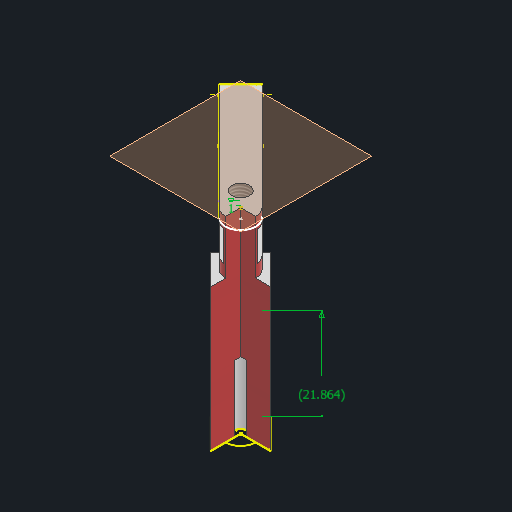
# Autodesk Inventor part: Redesign_Gripper_Finger
Saved by Autodesk Inventor 2025.1 (Build 291241000, 241)
## iProperties
Created: 2024-12-20
Part Number: Redesign_Gripper_Finger
Material: Generic
Document SubType Name: Modeling
Designer: m_kni
Density: 1 g/cm^3
Appearance: Default
Finish1_Area: 560.021 mm^2
Finish1_Appearance: Red
Finish1_Process: Prime/Paint RAL 3018
Finish1_Description: Prime/Paint RAL 3018
Finish1_ShortDescription: RAL 3018
Finish1_Thickness: 0.050 mm
Author: m_kni
## iProperties of the stored document Redesign_Gripper_Finger_3DPrint.ipt
Created: 2025-01-24
Part Number: Redesign_Gripper_Finger_3DPrint
Material: Generic
Document SubType Name: Modeling
Designer: m_kni
Density: 1 g/cm^3
Appearance: Default
Author: m_kni
Autodesk Inventor part; units mm, degrees
ref_plane "YZ Plane" through (0, 0, 0) normal (1, 0, 0) x (0, 1, 0)
ref_plane "XZ Plane" through (0, 0, 0) normal (0, 1, 0) x (-1, 0, 0)
ref_plane "XY Plane" through (0, 0, 0) normal (0, 0, 1) x (1, 0, 0)
sketch "Sketch1" plane through (0, 0, 0) normal (0, 1, 0) x (-1, 0, 0)
  arc A0 (-2.54, 0) -> (0, 2.54) centre (0, 0) ccw
  line L0 (0, 2.54) -> (0, 0)
  line L1 (0, 0) -> (-2.54, 0)
  dimension "d0" = 5.08
  constraints: 4 end point, 2 point on circle, 1 centre point, 1 coincident, 1 perpendicular, 1 vertical
  measures "d0" diameter of A0
extrude "Extrusion1" add sketch "Sketch1" along normal blind 25.4
sketch "Sketch2" plane through (0, 25.4, 0) normal (0, 1, 0) x (1, 0, 0)
  line L0 (0, -2.54) -> (0, 0) projected
  line L1 (0, 0) -> (-17.9605, 17.9605)
  line L2 (0, 0) -> (25.4, 0) construction
  line L3 (0, 0) -> (-1.7961, -1.7961)
  arc A0 (2.54, 0) -> (0, -2.54) centre (0, 0) ccw projected
  line L4 (0, 0) -> (1.7961, 1.7961)
  line L5 (-1.7961, -1.7961) -> (-19.7566, 16.1645)
  line L6 (-19.7566, 16.1645) -> (-17.9605, 17.9605)
  line L7 (-16.1645, 19.7566) -> (1.7961, 1.7961)
  line L8 (-16.1645, 19.7566) -> (-17.9605, 17.9605)
  line L9 (0, 0) -> (2.54, 0)
  dimension "d3" = 25.4
  dimension "d4" = 135
  constraints: 18 end point, 4 perpendicular, 3 point on circle, 2 horizontal, 2 point on line, 1 equal length, 1 tangent
  measures "d3" distance of L0.end L1.end
  measures "d4" angle of L2 L1
extrude "Extrusion2" add sketch "Sketch2" along normal blind 6
sketch "Sketch3" plane through (-19.7566, 25.4, -16.1645) normal (-0.7071068, 0, -0.7071068) x (-0.7071068, 0, 0.7071068)
  line L0 (-5.08, 0) -> (-5.08, 6) projected
  line L1 (0, 6) -> (-5.08, 6)
  line L2 (-5.08, 6) -> (-5.08, 0)
  line L3 (-5.08, 0) -> (0, 0)
  line L4 (0, 0.5) -> (0, 5.5)
  line L5 (-2.54, 6) -> (-4.3361, 6) projected
  line L6 (-2.54, 6) -> (-2.54, 0)
  line L7 (-4.54, 0) -> (-0.54, 0)
  line L8 (-0.54, 0.5) -> (-0.54, 5.5)
  line L9 (-0.54, 6) -> (-4.54, 6)
  line L10 (-4.54, 6) -> (-4.54, 0)
  line L11 (-4.54, 0) -> (-0.54, 6) construction
  line L12 (-0.54, 0) -> (-4.54, 6) construction
  line L13 (0, 0.5) -> (-5.08, 0.5)
  line L14 (-5.08, 0.5) -> (-5.08, 5.5)
  line L15 (-5.08, 5.5) -> (0, 5.5)
  line L16 (0, 0.5) -> (-5.08, 5.5) construction
  line L17 (-5.08, 0.5) -> (0, 5.5) construction
  line L18 (-5.08, 0) -> (0, 0)
  line L19 (0, 0) -> (0, 6)
  line L20 (0, 6) -> (-5.08, 6)
  line L21 (-5.08, 6) -> (-5.08, 0)
  line L22 (-5.08, 0) -> (0, 6) construction
  line L23 (0, 0) -> (-5.08, 6) construction
  line L24 (-0.7439, 6) -> (0, 6)
  line L25 (-5.08, 0) -> (0, 0)
  line L26 (0, 0) -> (0, 6)
  line L27 (0, 6) -> (-5.08, 6)
  line L28 (-5.08, 6) -> (-5.08, 0)
  line L29 (-5.08, 0) -> (0, 6) construction
  line L30 (0, 0) -> (-5.08, 6) construction
  line L31 (0, 6) -> (0, 0)
  line L32 (-4.54, 5.5) -> (-9.54, 5.5)
  line L33 (-9.54, 5.5) -> (-9.54, 0.5)
  line L34 (-9.54, 0.5) -> (-4.54, 0.5)
  line L35 (-4.54, 0.5) -> (-4.54, 5.5)
  line L36 (-0.54, 5.5) -> (4.46, 5.5)
  line L37 (4.46, 5.5) -> (4.46, 0.5)
  line L38 (4.46, 0.5) -> (-0.54, 0.5)
  line L39 (-0.54, 0.5) -> (-0.54, 5.5)
  point P0 (-2.54, -25.4)
  point P1 (-2.54, 3)
  point P2 (-4.54, 5.5)
  point P3 (-5.08, 5.5)
  point P4 (-5.08, 0.5)
  point P5 (-4.54, 0.5)
  point P6 (0, 5.5)
  point P7 (0, 0.5)
  point P8 (-5.08, 0.5)
  point P9 (-5.08, 5.5)
  dimension "d7" = 4
  dimension "d8" = 5
  dimension "d11" = 6
  dimension "d40" = 5
  dimension "d41" = 5
  constraints: 76 end point, 13 parallel, 10 midpoint, 7 horizontal, 7 perpendicular, 7 point on line, 1 collinear, 1 vertical
  measures "d7" distance of L9.end L9.start
  measures "d8" distance of L13.end L14.end
  measures "d11" distance of L0.start L1.end
  measures "d40" distance of L34.end L33.end
  measures "d41" distance of L37.end L38.end
extrude "Extrusion5" cut sketch "Sketch3" against normal blind 33.8125 contours L34 L33 L32 L0 | L0 L15 L10 L13 | L8 L15 L4 L13 | L4 L36 L37 L38
sketch "Sketch6" plane through (0, 31.4, 0) normal (0, 1, 0) x (1, 0, 0)
  arc A0 (1.7961, 1.7961) -> (-1.7961, -1.7961) centre (0, 0) ccw projected
  circle A1 centre (0, 0) radius 2.54
  line L0 (1.7961, 1.7961) -> (-16.1645, 19.7566) projected
  line L1 (0, 3.5921) -> (-3.5921, 0)
  line L2 (-19.7566, 16.1645) -> (-1.7961, -1.7961) projected
  line L3 (-1.7961, 1.7961) -> (-2.5032, 2.5032)
  circle A2 centre (-2.5032, 2.5032) radius 2.54
  dimension "d16" = 1
  constraints: 4 end point, 2 coincident, 2 point on line, 1 centre point, 1 midpoint, 1 tangent, 3 other
  measures "d16" distance of L3.start L3.end
ref_plane "Work Plane3" through (-2.5032, 37.9, -2.5032) normal (0, 1, 0) x (1, 0, 0)
sketch "Sketch7" plane through (-2.5032, 37.9, -2.5032) normal (0, 1, 0) x (1, 0, 0)
  circle A0 centre (0, 0) radius 1.5
  point P0 (2.5032, -2.5032)
  dimension "d19" = 3
  constraints: 1 centre point
  measures "d19" diameter of A0
extrude "Extrusion7" cut sketch "Sketch7" against normal blind 6
sketch "Sketch10" plane through (0, 31.4, 0) normal (0, 1, 0) x (1, 0, 0)
  arc A0 (-1.7961, -1.7961) -> (0, -2.54) centre (0, 0) ccw projected
  line L0 (0, -2.54) -> (0, 0) projected
  line L1 (0, 0) -> (2.54, 0) projected
  line L2 (1.7961, 1.7961) -> (-16.1645, 19.7566) projected
  line L3 (-19.7566, 16.1645) -> (-1.7961, -1.7961) projected
  line L4 (-19.7566, 16.1645) -> (-1.7961, -1.7961) projected
  line L5 (-16.1645, 19.7566) -> (-19.7566, 16.1645) projected
  line L6 (1.7961, 1.7961) -> (-16.1645, 19.7566) projected
  arc A1 (2.54, 0) -> (1.7961, 1.7961) centre (0, 0) ccw projected
  point P0 (-0.7071, 4.2992)
  point P1 (2.5214, 0.3071)
  point P2 (-4.2992, 0.7071)
extrude "Extrusion9" add sketch "Sketch10" along normal blind 1.5
sketch "Sketch11" plane through (0, 25.4, 0) normal (0, -1, 0) x (1, 0, 0)
  arc A0 (-1.7961, 1.7961) -> (1.7961, -1.7961) centre (0, 0) ccw projected
  line L0 (-19.7566, -16.1645) -> (-1.7961, 1.7961) projected
  line L1 (-16.1645, -19.7566) -> (-19.7566, -16.1645) projected
  line L2 (1.7961, -1.7961) -> (-16.1645, -19.7566) projected
extrude "Extrusion10" add sketch "Sketch11" along normal blind 1.5
sketch "Sketch13" plane through (0, 0, 0) normal (0, -1, 0) x (1, 0, 0)
  line L0 (0, 0) -> (2.54, 0) projected
  arc A0 (0, 5) -> (5, 0) centre (0, 0) ccw
  line L1 (0, 0) -> (0, 5)
  line L2 (0, 0) -> (5, 0)
  dimension "d37" = 10
  constraints: 4 end point, 2 point on circle, 1 centre point, 1 coincident, 1 perpendicular, 1 vertical
  measures "d37" diameter of A0
extrude "Extrusion12" add sketch "Sketch13" against normal up to surface (23.9 mm away)
sketch "Sketch14" plane through (0, 0, 0) normal (0, -1, 0) x (1, 0, 0)
  circle A0 centre (0, 0) radius 1
  dimension "d42" = 2
  constraints: 1 centre point, 1 coincident
  measures "d42" diameter of A0
extrude "Extrusion13" cut sketch "Sketch14" against normal blind 11.2
sketch "Sketch15" plane through (0, 32.9, 0) normal (0, 1, 0) x (1, 0, 0)
  circle A0 centre (-2.5032, 2.5032) radius 1.5 projected
  circle A1 centre (-2.5032, 2.5032) radius 1.5
  point P0 (0, 0)
  constraints: 1 centre point, 1 coincident, 1 concentric
extrude "Extrusion14" cut sketch "Sketch15" against normal blind 8
thread "Thread2" size "M3x0.5" class "6H" standard "ANSI Metric M Profile" full length
sketch "Sketch16" plane through (0, 0, 0) normal (0, -1, 0) x (1, 0, 0)
  arc A0 (0, 5) -> (5, 0) centre (0, 0) ccw projected
  line L0 (0, 0) -> (3.981, 3.981)
  line L1 (0, 0) -> (5.63, 0) construction
  line L2 (0, 5) -> (-5, 0)
  line L3 (5, 0) -> (0, -5)
  line L4 (-5, 0) -> (0, -5)
  circle A1 centre (0, 0) radius 5
  dimension "d52" = 45
  constraints: 10 end point, 5 point on circle, 1 centre point, 1 coincident, 1 equal length, 1 horizontal
  measures "d52" angle of L1 L0
extrude "Extrusion15" cut sketch "Sketch16" against normal up to surface (23.9 mm away) contours L2 A0 | L4 A0 | L3 A0
sketch "Sketch17" plane through (-19.3747, 25.9, -16.5463) normal (-0.7071068, 0, -0.7071068) x (-0.7071068, 0, 0.7071068)
  line L0 (0, 0) -> (0.54, 0) projected
  line L1 (0.54, 5) -> (0, 5) projected
  line L2 (-4, 0) -> (-4, 5) projected
  line L3 (-4.54, 0) -> (-4, 0) projected
  line L4 (-4, 5) -> (-4.54, 5) projected
  line L5 (0.54, -2) -> (0.54, 0) projected
  line L6 (0.54, -2) -> (-0.2039, -2) projected
  line L7 (-2, 7) -> (-3.7961, 7) projected
  line L8 (-4.54, 5) -> (-4.54, 7) projected
  line L9 (-3.7961, 7) -> (-4.54, 7) projected
  line L10 (0.54, -2) -> (-0.2039, -2) projected
  line L11 (-0.2039, -2) -> (-0.2039, 7) projected
  line L12 (0.54, 7) -> (-0.2039, 7) projected
  line L13 (0.54, 5) -> (0.54, 7) projected
  line L14 (0.54, 5) -> (0, 5) projected
  line L15 (0, 5) -> (0, 0) projected
  line L16 (0, 0) -> (0.54, 0) projected
  line L17 (0.54, -2) -> (0.54, 0) projected
  line L18 (-3.7961, -2) -> (-3.7961, 7) projected
  line L19 (-3.7961, -2) -> (-4.54, -2) projected
  line L20 (-4.54, -2) -> (-4.54, 0) projected
  line L21 (-4.54, 0) -> (-4, 0) projected
  line L22 (-4, 0) -> (-4, 5) projected
  line L23 (-4, 5) -> (-4.54, 5) projected
  line L24 (-4.54, 5) -> (-4.54, 7) projected
  line L25 (-3.7961, 7) -> (-4.54, 7) projected
  line L26 (-3.7961, -2) -> (-3.7961, 7) projected
  line L27 (0.54, -2) -> (-4.54, -2) projected
  line L28 (0, 5) -> (0, 0) projected
  line L29 (-3.7961, -2) -> (-4.54, -2) projected
  line L30 (0.54, -2) -> (-4.54, -2) projected
  line L31 (0.54, 0) -> (0, 0) projected
  line L32 (0, 0) -> (0, 5) projected
  line L33 (0, 5) -> (0.54, 5) projected
  line L34 (0.54, 5) -> (0.54, 7) projected
  line L35 (-4.54, 7) -> (0.54, 7) projected
  line L36 (-4.54, 5) -> (-4.54, 7) projected
  line L37 (-4.54, 5) -> (-4, 5) projected
  line L38 (-4, 5) -> (-4, 0) projected
  line L39 (-4, 0) -> (-4.54, 0) projected
  line L40 (-4.54, -2) -> (-4.54, 0) projected
  line L41 (0.54, -2) -> (-4.54, -2) projected
  line L42 (0.54, 0) -> (0.54, -2) projected
  line L43 (-3.5, 7) -> (-0.5, 7) projected
  line L44 (-0.2039, 7) -> (-2, 7) projected
  line L45 (-2, 7) -> (-3.7961, 7) projected
  line L46 (-3.7961, 7) -> (-4.54, 7) projected
  line L47 (-4.54, 7) -> (0.54, 7) projected
  line L48 (0.54, 7) -> (-0.2039, 7) projected
  line L49 (0.54, -2) -> (-4.54, -2) projected
  line L50 (0.54, -2) -> (-4.54, -2) projected
  line L51 (0.54, 5) -> (0.54, 7) projected
  line L52 (0, 5) -> (0.54, 5) projected
  line L53 (0.54, 5) -> (0.54, 7) projected
  line L54 (0.54, 0) -> (0, 0) projected
  line L55 (0.54, 5) -> (0.54, 7) projected
  line L56 (0.54, 5) -> (0.54, 7) projected
  line L57 (0.54, 0) -> (0.54, -2) projected
  line L58 (0.54, -2) -> (0.54, 0) projected
  line L59 (0.54, 5) -> (0, 5) projected
  line L60 (0, 5) -> (0.54, 5) projected
  line L61 (0, 0) -> (0.54, 0) projected
  line L62 (0.54, 0) -> (0, 0) projected
  line L63 (0, 5) -> (0, 0) projected
  line L64 (0, 0) -> (0, 5) projected
  line L65 (-4.54, -2) -> (-4.54, 0) projected
  line L66 (0.54, 7) -> (-0.2039, 7) projected
  line L67 (-4.54, 5) -> (-4.54, 7) projected
  line L68 (-4.54, -2) -> (-4.54, 0) projected
  line L69 (-4, 0) -> (-4.54, 0) projected
  line L70 (-4.54, 5) -> (-4, 5) projected
  line L71 (-4, 0) -> (-4, 5) projected
  line L72 (-4, 5) -> (-4, 0) projected
  line L73 (-4, 0) -> (-4.54, 0) projected
  line L74 (-4.54, 0) -> (-4, 0) projected
  line L75 (-4, 5) -> (-4.54, 5) projected
  line L76 (-4.54, 5) -> (-4, 5) projected
  line L77 (-4.54, -2) -> (-4.54, 0) projected
  line L78 (-4.54, -2) -> (-4.54, 0) projected
  line L79 (-4.54, 5) -> (-4.54, 7) projected
  line L80 (-4.54, 5) -> (-4.54, 7) projected
  line L81 (-4.54, 7) -> (0.54, 7) projected
  line L82 (-4, 5) -> (-4, 0) projected
  line L83 (0.54, 0) -> (0.54, -2) projected
  line L84 (-0.2039, -2) -> (-0.2039, 7) projected
  line L85 (-3.5, -1) -> (-0.5, -1) projected
  line L86 (-3.5, -1) -> (-0.5, -1) projected
  line L87 (-3.5, 7) -> (-0.5, 7) projected
  line L88 (-3.5, -1) -> (-0.5, -1) projected
  line L89 (-3.5, 7) -> (-0.5, 7) projected
  line L90 (0, 0) -> (0, 5) projected
  line L91 (-0.2039, 7) -> (-2, 7) projected
  line L92 (0.54, 5.5) -> (-4.54, 5.5) projected
  line L93 (0.54, 5.5) -> (-4.54, 5.5) projected
  line L94 (-4.54, 5.5) -> (0.54, 5.5) projected
  line L95 (0.54, 5.5) -> (-4.54, 5.5) projected
  point P0 (-2, -25.9)
  point P1 (-2, 5.5)
  point P2 (-2, 5.5)
  point P3 (-2, 5.5)
  point P4 (-4.54, 5.5)
  point P5 (0.54, 5.5)
  point P6 (0.54, 5.5)
  point P7 (-2, 5.5)
  point P8 (-2, 5.5)
  point P9 (-2, 5.5)
  point P10 (-2, 5.5)
  constraints: 8 other
sketch "Sketch18" plane through (0, 32.9, 0) normal (0, 1, 0) x (1, 0, 0)
  point P0 (0, 0)
sketch "Sketch19" plane through (0, 0, 0) normal (0, -1, 0) x (1, 0, 0)
  arc A0 (-0.3071, 2.5214) -> (-1.7961, 1.7961) centre (0, 0) ccw projected
  arc A1 (-0.3071, 2.5214) -> (-1.7961, 1.7961) centre (0, 0) ccw projected
  arc A2 (1.7961, -1.7961) -> (2.5214, -0.3071) centre (0, 0) ccw projected
  arc A3 (1.7961, -1.7961) -> (2.5214, -0.3071) centre (0, 0) ccw projected
  arc A4 (0, 2.54) -> (-1.7961, 1.7961) centre (0, 0) ccw projected
  line L0 (0, 5) -> (0, 2.54) projected
  line L1 (0, 0) -> (2.54, 0) projected
  line L2 (-1.7961, 1.7961) -> (-4.2961, -0.7039) projected
  arc A5 (1.7961, -1.7961) -> (2.54, 0) centre (0, 0) ccw projected
  line L3 (-4.2961, -0.7039) -> (-5, 0) projected
  arc A6 (0, 2.54) -> (-1.7961, 1.7961) centre (0, 0) ccw projected
  arc A7 (0, 2.54) -> (-1.7961, 1.7961) centre (0, 0) ccw projected
  arc A8 (-0.3071, 2.5214) -> (-1.7961, 1.7961) centre (0, 0) ccw projected
  arc A9 (-0.3071, 2.5214) -> (-1.7961, 1.7961) centre (0, 0) ccw projected
  line L4 (-5, 0) -> (0, 5) projected
  line L5 (-5, 0) -> (0, 5) projected
  line L6 (0, 5) -> (0, 2.54) projected
  arc A10 (0, 2.54) -> (-1.7961, 1.7961) centre (0, 0) ccw projected
  line L7 (-1.7961, 1.7961) -> (-4.2961, -0.7039) projected
  line L8 (-4.2961, -0.7039) -> (-5, 0) projected
  arc A11 (1.7961, -1.7961) -> (2.54, 0) centre (0, 0) ccw projected
  arc A12 (1.7961, -1.7961) -> (2.5214, -0.3071) centre (0, 0) ccw projected
  arc A13 (1.7961, -1.7961) -> (2.5214, -0.3071) centre (0, 0) ccw projected
  arc A14 (1.7961, -1.7961) -> (2.54, 0) centre (0, 0) ccw projected
  line L9 (-4.2961, -0.7039) -> (-0.7039, -4.2961) projected
  line L10 (0, 1) -> (0, 0) projected
  line L11 (0, 1) -> (0, 0) projected
  line L12 (0, 2.54) -> (0, 0) projected
  line L13 (0, 5) -> (0, 2.54) projected
  line L14 (0, 5) -> (0, 1) projected
  line L15 (0, 0) -> (1, 0) projected
  line L16 (1, 0) -> (5, 0) projected
  line L17 (2.54, 0) -> (5, 0) projected
  line L18 (0, 0) -> (2.54, 0) projected
  line L19 (5, 0) -> (0, -5) projected
  line L20 (0, -5) -> (5, 0) projected
  line L21 (-4.2961, -0.7039) -> (-5, 0) projected
  line L22 (-4.2961, -0.7039) -> (-0.7039, -4.2961) projected
  line L23 (0, -5) -> (-0.7039, -4.2961) projected
  line L24 (-5, 0) -> (0, -5) projected
  line L25 (-5, 0) -> (0, -5) projected
  line L26 (0, 5) -> (-5, 0) projected
  line L27 (-5, 0) -> (0, 5) projected
  line L28 (0, 5) -> (-5, 0) projected
  line L29 (0, -5) -> (-0.7039, -4.2961) projected
  arc A15 (1.7961, -1.7961) -> (2.54, 0) centre (0, 0) ccw projected
  line L30 (-0.7039, -4.2961) -> (1.7961, -1.7961) projected
  line L31 (2.54, 0) -> (5, 0) projected
  line L32 (5, 0) -> (0, -5) projected
  line L33 (0, -5) -> (-0.7039, -4.2961) projected
  line L34 (-0.7039, -4.2961) -> (1.7961, -1.7961) projected
  arc A16 (1.7961, -1.7961) -> (2.54, 0) centre (0, 0) ccw projected
  line L35 (2.54, 0) -> (5, 0) projected
  line L36 (5, 0) -> (0, -5) projected
  arc A17 (0, 2.54) -> (-1.7961, 1.7961) centre (0, 0) ccw projected
  circle A18 centre (-2.5032, -2.5032) radius 1.5 projected
  circle A19 centre (-2.5032, -2.5032) radius 1.5 projected
  circle A20 centre (-2.5032, -2.5032) radius 1.5 projected
  circle A21 centre (-2.5032, -2.5032) radius 1.5 projected
  circle A22 centre (-2.5032, -2.5032) radius 1.5 projected
  line L37 (0, 5) -> (0, 1) projected
  arc A23 (0, 1) -> (1, 0) centre (0, 0) ccw projected
  line L38 (0, -5) -> (5, 0) projected
  line L39 (1, 0) -> (5, 0) projected
  line L40 (0, 0) -> (1, 0) projected
  arc A24 (0, 1) -> (1, 0) centre (0, 0) ccw projected
  line L41 (0, 0) -> (1, 0) projected
  line L42 (0, 1) -> (0, 0) projected
  arc A25 (0, 1) -> (1, 0) centre (0, 0) ccw projected
  arc A26 (0, 1) -> (1, 0) centre (0, 0) ccw projected
  arc A27 (0, 1) -> (1, 0) centre (0, 0) ccw projected
  line L43 (0, 5) -> (-5, 0) projected
  line L44 (-5, 0) -> (0, -5) projected
  line L45 (0, -5) -> (5, 0) projected
  line L46 (1, 0) -> (5, 0) projected
  arc A28 (0, 1) -> (1, 0) centre (0, 0) ccw projected
  line L47 (0, 5) -> (0, 1) projected
  line L48 (0, 2.54) -> (0, 0) projected
  arc A29 (-1.7961, 1.7961) -> (1.7961, -1.7961) centre (0, 0) ccw projected
  circle A30 centre (0, 0) radius 2.54 projected
  line L49 (0, -3.5921) -> (-3.5921, 0) projected
  line L50 (-1.7961, -1.7961) -> (-2.5032, -2.5032) projected
  circle A31 centre (-2.5032, -2.5032) radius 2.54 projected
  line L51 (-19.7566, -16.1645) -> (-16.1645, -19.7566) projected
  dimension "d55" = 21.8645
  constraints: 12 other
  measures "d55" distance between parallel lines of L9 L51
body "Solid1"
